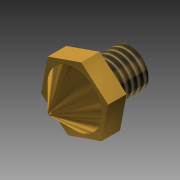
# Autodesk Inventor part: heNozzle
Saved by Autodesk Inventor 2013 (Build 170138000, 138)
## iProperties
Created: 2015-01-15
Part Number: heNozzle
Material: Generic
Document SubType Name: Modeling
Designer: dzban
Density: 1 g/cm^3
Author: dzban
Autodesk Inventor part; units mm, degrees
ref_plane "YZ Plane" through (0, 0, 0) normal (1, 0, 0) x (0, 1, 0)
ref_plane "XZ Plane" through (0, 0, 0) normal (0, 1, 0) x (-1, 0, 0)
ref_plane "XY Plane" through (0, 0, 0) normal (0, 0, 1) x (1, 0, 0)
sketch "Sketch1" plane through (0, 0, 0) normal (0, 0, 1) x (1, 0, 0)
  line L0 (0.2, 0) -> (0.2, 1)
  line L1 (0.2, 1) -> (1, 1.5292)
  line L2 (1, 1.5292) -> (1, 13)
  line L3 (1, 13) -> (3, 13)
  line L4 (3, 13) -> (3, 7)
  line L5 (3, 7) -> (9, 7)
  line L6 (9, 7) -> (9, 4)
  line L7 (9, 4) -> (4.4, 4)
  line L8 (4.4, 4) -> (0.4, 0)
  line L9 (0.4, 0) -> (0.2, 0)
  line L10 (0, 0) -> (0, 2.7368)
  dimension "d0" = 0.2
  dimension "d2" = 0.4
  dimension "d4" = 45
  dimension "d5" = 1
  dimension "d6" = 3
  dimension "d7" = 9
  dimension "d8" = 13
  dimension "d9" = 3
  dimension "d10" = 4
  dimension "d11" = 1
  constraints: 22 end point, 4 horizontal, 4 vertical, 1 horizontal alignment
  measures "d0" distance between parallel lines of L0 L10
  measures "d2" distance from line of L8.end L10
  measures "d4" angle of L8 L9
  measures "d5" distance between parallel lines of L2 L10
  measures "d6" distance between parallel lines of L4 L10
  measures "d7" distance between parallel lines of L6 L10
  measures "d8" distance between parallel lines of L3 L9
  measures "d9" distance between parallel lines of L5 L7
  measures "d10" distance between parallel lines of L7 L9
  measures "d11" distance from line of L0.end L9
revolve "Revolution1" add sketch "Sketch1" angle 360 about axis through (0, 0, 0) along (0, 1, 0)
sketch "Sketch2" plane through (0, 7, 0) normal (0, 1, 0) x (1, 0, 0)
  circle A0 centre (0, 0) radius 9 projected
  circle A1 centre (0, 0) radius 3 projected
  line L0 (1.0809, -5.6714) -> (-4.3711, -3.7718)
  line L1 (-4.3711, -3.7718) -> (-5.452, 1.8996)
  line L2 (-5.452, 1.8996) -> (-1.0809, 5.6714)
  line L3 (-1.0809, 5.6714) -> (4.3711, 3.7718)
  line L4 (4.3711, 3.7718) -> (5.452, -1.8996)
  line L5 (5.452, -1.8996) -> (1.0809, -5.6714)
  dimension "d13" = 10
  constraints: 12 end point, 1 coincident, 13 other
  measures "d13" distance between parallel lines of L3 L0
extrude "Extrusion1" cut sketch "Sketch2" against normal blind 10 contours A0
thread "Thread1" size "M6x1" class "6g" standard "ANSI Metric M Profile" full length
body "Solid1"
